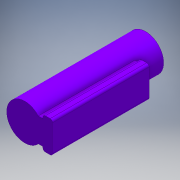
# Autodesk Inventor part: flat_cover_5mm
Saved by Autodesk Inventor 2018 (Build 220112000, 112)
## iProperties
Created: 2019-01-24
Part Number: flat_cover_5mm
Material: 一般
Document SubType Name: Modeling
Designer: lowyu
Density: 1 g/cm^3
Appearance: 既定
Author: lowyu
## iProperties of the stored document flat_cover_5mm_3D プリント.ipt
Created: 2019-01-24
Part Number: flat_cover_5mm_3D プリント
Material: 一般
Document SubType Name: Modeling
Designer: lowyu
Density: 1 g/cm^3
Appearance: 既定
Author: lowyu
Autodesk Inventor part; units mm, degrees
ref_plane "YZ Plane" through (0, 0, 0) normal (1, 0, 0) x (0, 1, 0)
ref_plane "XZ Plane" through (0, 0, 0) normal (0, 1, 0) x (-1, 0, 0)
ref_plane "XY Plane" through (0, 0, 0) normal (0, 0, 1) x (1, 0, 0)
sketch "スケッチ1" plane through (0, 0, 0) normal (0, 0, 1) x (1, 0, 0)
  line L0 (0, 25) -> (-3.75, 25)
  line L1 (-3.75, 25) -> (-3.75, 0)
  line L2 (-3.75, 0) -> (0, 0)
  line L3 (0, 0) -> (0, 25)
  line L4 (0, -5) -> (0, 30) projected
  line L5 (-4.5, 0) -> (0.75, 0) projected
  dimension "d2" = 3.75
  dimension "d3" = 25
  constraints: 8 end point, 2 collinear, 2 parallel, 1 horizontal, 1 perpendicular
  measures "d2" distance of L2.end L1.end
  measures "d3" distance of L1.end L0.end
revolve "回転1" add sketch "スケッチ1" angle 360 about axis through (0, -10, 0) along (0, 1, 0)
sketch "スケッチ3" plane through (0, 25, 0) normal (0, 1, 0) x (1, 0, 0)
  circle A0 centre (0, 0) radius 2.525
  dimension "d5" = 5.05
  constraints: 1 centre point, 1 coincident
  measures "d5" diameter of A0
extrude "押し出し1" cut sketch "スケッチ3" against normal blind 5
sketch "スケッチ4" plane through (0, 0, 0) normal (0, -1, 0) x (1, 0, 0)
  circle A0 centre (0, 0) radius 3.75 projected
  line L0 (3.75, 3.25) -> (5.75, 3.25)
  line L1 (3.75, -3.25) -> (5.75, -3.25)
  line L2 (5.75, -3.25) -> (5.75, 3.25)
  line L3 (2.7951, 2.5) -> (3.75, 2.5)
  line L4 (-5.65, 0) -> (7.65, 0) projected
  line L5 (3.75, 3.25) -> (3.75, 2.5)
  line L6 (3.75, 0) -> (3.75, -3.25)
  line L7 (2.7951, -2.5) -> (3.75, -2.5)
  dimension "d9" = 6.5
  dimension "d10" = 2
  dimension "d11" = 2.5
  dimension "d12" = 5
  constraints: 14 end point, 4 perpendicular, 2 horizontal, 2 point on circle, 2 point on line, 2 tangent, 2 vertical
  measures "d9" distance of L0.start L1.start
  measures "d10" distance of L0.start L0.end
  measures "d11" distance between parallel lines of L4 L3
  measures "d12" distance between parallel lines of L7 L3
extrude "押し出し2" add sketch "スケッチ4" against normal blind 20 contours L6 L7 A0 | A0 L3 L5 L0 L2 L4 | L4 L2 L1 L6
fillet "フィレット1" radius 0.5 4 edges at (5.75, 10, 3.25) (5.75, 10, -3.25) (3.75, 10, 3.25) (3.75, 10, -3.25)
